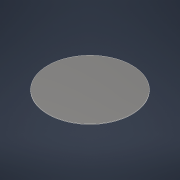
# Autodesk Inventor part: McCrea_ukruhlaPlocha_walle
Saved by Autodesk Inventor 2022 (Build 260153000, 153)
## iProperties
Created: 2022-02-09
Part Number: McCrea_ukruhlaPlocha_walle
Material: Rubber
Document SubType Name: Modeling
Designer: MatusBarany
Density: 0.93 g/cm^3
Appearance: Rubber - Black
Author: MatusBarany
Autodesk Inventor part; units mm, degrees
ref_plane "YZ Plane" through (0, 0, 0) normal (1, 0, 0) x (0, 1, 0)
ref_plane "XZ Plane" through (0, 0, 0) normal (0, 1, 0) x (-1, 0, 0)
ref_plane "XY Plane" through (0, 0, 0) normal (0, 0, 1) x (1, 0, 0)
sketch "Sketch1" plane through (0, 0, 0) normal (0, 1, 0) x (-1, 0, 0)
  circle A0 centre (0, 0) radius 850
  dimension "d0" = 1700
  constraints: 1 centre point, 1 coincident
  measures "d0" diameter of A0
extrude "Extrusion1" add sketch "Sketch1" along normal blind 10
sketch "Sketch2" plane through (0, 0, 0) normal (0, -1, 0) x (1, 0, 0)
  circle A0 centre (0, 0) radius 2.5
  dimension "d3" = 5
  constraints: 1 centre point, 1 coincident
  measures "d3" diameter of A0
extrude "Extrusion2" cut sketch "Sketch2" against normal blind 5
sketch "Sketch3" plane through (0, 0, 0) normal (0, -1, 0) x (1, 0, 0)
  line L0 (-114.2279, 383.8588) -> (126.182, 383.8588)
  line L1 (126.182, 383.8588) -> (126.182, 257.6769)
  line L2 (126.182, 257.6769) -> (-114.2279, 257.6769)
  line L3 (-114.2279, 257.6769) -> (-114.2279, 383.8588)
  point P0 (0, 0)
  constraints: 8 end point, 2 parallel, 1 horizontal, 1 perpendicular
extrude "Extrusion3" add sketch "Sketch3" along normal blind 5
body "Solid1"
